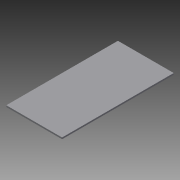
# Autodesk Inventor part: MainBoard
Saved by Autodesk Inventor 2015 SP2 (Build 190223200, 223)
## iProperties
Created: 2016-03-22
Part Number: MainBoard
Material: Generic
Document SubType Name: Modeling
Designer: cvhssub1
Density: 1 g/cm^3
Appearance: Default
Author: cvhssub1
Autodesk Inventor part; units mm, degrees
ref_plane "YZ Plane" through (0, 0, 0) normal (1, 0, 0) x (0, 1, 0)
ref_plane "XZ Plane" through (0, 0, 0) normal (0, 1, 0) x (-1, 0, 0)
ref_plane "XY Plane" through (0, 0, 0) normal (0, 0, 1) x (1, 0, 0)
sketch "Sketch1" plane through (0, 0, 0) normal (0, 1, 0) x (-1, 0, 0)
  line L0 (0, 0) -> (12, 0)
  line L1 (12, 0) -> (12, -30)
  line L2 (12, -30) -> (0, -30)
  line L3 (0, -30) -> (0, 0)
  dimension "d0" = 12
  constraints: 8 end point, 2 parallel, 1 horizontal, 1 perpendicular
  measures "d0" distance of L1.end L2.end
extrude "Extrusion1" add sketch "Sketch1" along normal blind 0.2
sketch "Sketch2" plane through (0, 0.2, 0) normal (0, 1, 0) x (1, 0, 0)
  line L0 (0, 30) -> (0, -1.3153) construction
  line L1 (0, -1.3153) -> (-12, -1.3153) construction
  line L2 (-12, -1.3153) -> (-12, 30) construction
  line L3 (-12, 30) -> (0, 30) construction
  line L4 (0, 0) -> (0, 30) projected
  line L5 (0, 30) -> (-12, 30) projected
  line L6 (-12, 30) -> (-12, 0)
  line L7 (-12, 30) -> (-12, 0) projected
  dimension "d20" = 0
  dimension "d23" = 0
  constraints: 2 end point, 1 point on line, 2 other
  measures "d20" distance between parallel lines of L0 L4
  measures "d23" distance between parallel lines of L5 L3
body "Solid1"
